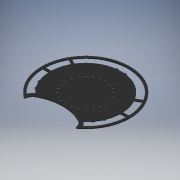
# Autodesk Inventor part: MotorPlate
Saved by Autodesk Inventor 2017 (Build 210142000, 142)
## iProperties
Created: 2019-01-31
Part Number: MotorPlate
Material: Generic
Document SubType Name: Modeling
Designer: cresswnd
Density: 1 g/cm^3
Appearance: Smooth - Black
Author: cresswnd
Autodesk Inventor part; units mm, degrees
ref_plane "YZ Plane" through (0, 0, 0) normal (1, 0, 0) x (0, 1, 0)
ref_plane "XZ Plane" through (0, 0, 0) normal (0, 1, 0) x (-1, 0, 0)
ref_plane "XY Plane" through (0, 0, 0) normal (0, 0, 1) x (1, 0, 0)
sketch "Sketch1" plane through (0, 0, 0) normal (0, 1, 0) x (-1, 0, 0)
  circle A0 centre (0, 0) radius 13.5 construction
  circle A1 centre (0, 0) radius 43
  line L0 (0, 0) -> (0, 137) construction
  line L1 (0, 43) -> (0, 47.5) construction
  circle A2 centre (0, 47.5) radius 2.5
  circle A3 centre (-6.2, 47.0936) radius 2.5
  circle A4 centre (-12.2939, 45.8815) radius 2.5
  circle A5 centre (-18.1775, 43.8843) radius 2.5
  circle A6 centre (-23.75, 41.1362) radius 2.5
  circle A7 centre (-28.9162, 37.6843) radius 2.5
  circle A8 centre (-33.5876, 33.5876) radius 2.5
  circle A9 centre (-37.6843, 28.9162) radius 2.5
  circle A10 centre (-41.1362, 23.75) radius 2.5
  circle A11 centre (-43.8843, 18.1775) radius 2.5
  circle A12 centre (-45.8815, 12.2939) radius 2.5
  circle A13 centre (-47.0936, 6.2) radius 2.5
  circle A14 centre (-47.5, 0) radius 2.5
  circle A15 centre (-47.0936, -6.2) radius 2.5
  circle A16 centre (-45.8815, -12.2939) radius 2.5
  circle A17 centre (-43.8843, -18.1775) radius 2.5
  circle A18 centre (-41.1362, -23.75) radius 2.5
  circle A19 centre (-37.6843, -28.9162) radius 2.5
  circle A20 centre (-33.5876, -33.5876) radius 2.5
  circle A21 centre (-28.9162, -37.6843) radius 2.5
  circle A22 centre (-23.75, -41.1362) radius 2.5
  circle A23 centre (-18.1775, -43.8843) radius 2.5
  circle A24 centre (-12.2939, -45.8815) radius 2.5
  circle A25 centre (-6.2, -47.0936) radius 2.5
  circle A26 centre (0, -47.5) radius 2.5
  circle A27 centre (6.2, -47.0936) radius 2.5
  circle A28 centre (12.2939, -45.8815) radius 2.5
  circle A29 centre (18.1775, -43.8843) radius 2.5
  circle A30 centre (23.75, -41.1362) radius 2.5
  circle A31 centre (28.9162, -37.6843) radius 2.5
  circle A32 centre (33.5876, -33.5876) radius 2.5
  circle A33 centre (37.6843, -28.9162) radius 2.5
  circle A34 centre (41.1362, -23.75) radius 2.5
  circle A35 centre (43.8843, -18.1775) radius 2.5
  circle A36 centre (45.8815, -12.2939) radius 2.5
  circle A37 centre (47.0936, -6.2) radius 2.5
  circle A38 centre (47.5, 0) radius 2.5
  circle A39 centre (47.0936, 6.2) radius 2.5
  circle A40 centre (45.8815, 12.2939) radius 2.5
  circle A41 centre (43.8843, 18.1775) radius 2.5
  circle A42 centre (41.1362, 23.75) radius 2.5
  circle A43 centre (37.6843, 28.9162) radius 2.5
  circle A44 centre (33.5876, 33.5876) radius 2.5
  circle A45 centre (28.9162, 37.6843) radius 2.5
  circle A46 centre (23.75, 41.1362) radius 2.5
  circle A47 centre (18.1775, 43.8843) radius 2.5
  circle A48 centre (12.2939, 45.8815) radius 2.5
  circle A49 centre (6.2, 47.0936) radius 2.5
  line L2 (0, 105) -> (0, 80) construction
  line L3 (0, 80) -> (-94, 80) construction
  line L4 (0, 80) -> (0, 55) construction
  line L5 (60, 80) -> (60, 65) construction
  line L6 (-60, 80) -> (-60, 65) construction
  line L7 (-60, 80) -> (-50, 80) construction
  line L8 (-50, 80) -> (-50, 65) construction
  line L9 (60, 80) -> (50, 80) construction
  line L10 (50, 80) -> (50, 65) construction
  arc A50 (-50, 67.6691) -> (50, 67.6691) centre (0, 160) ccw
  arc A51 (-60, 80) -> (-50, 67.6691) centre (-40.1315, 85.8924) ccw
  arc A52 (50, 67.6691) -> (60, 80) centre (40.1315, 85.8924) ccw
  circle A53 centre (-40.1315, 85.8924) radius 20.7239 construction
  circle A54 centre (40.1315, 85.8924) radius 20.7239 construction
  line L11 (0, 0) -> (0, -105) construction
  line L12 (0, 0) -> (105, 0) construction
  line L13 (0, 0) -> (105, 0) construction
  line L14 (0, 0) -> (-141, 0) construction
  line L15 (60, 0) -> (100, 0) construction
  line L16 (80, 0) -> (80, -2.5) construction
  line L17 (80, -2.5) -> (80, 2.5) construction
  line L18 (-60, 0) -> (-100, 0) construction
  line L19 (-80, 0) -> (-80, -2.5) construction
  line L20 (-80, -2.5) -> (-80, 2.5) construction
  line L21 (0, 0) -> (86.6025, 50) construction
  line L22 (0, 0) -> (100, 0) construction
  line L23 (0, 0) -> (-90.9327, 52.5) construction
  line L24 (0, 0) -> (105, 0) construction
  line L25 (-86.6025, 50) -> (-71.0141, 41) construction
  line L26 (-66.3266, 49.119) -> (-75.7016, 32.881) construction
  circle A55 centre (-66.3266, 49.119) radius 1.5 construction
  circle A56 centre (-66.3266, 49.119) radius 4 construction
  circle A57 centre (-75.7016, 32.881) radius 1.5 construction
  circle A58 centre (-75.7016, 32.881) radius 4 construction
  circle A59 centre (-75.7016, 32.881) radius 1.5
  circle A60 centre (-66.3266, 49.119) radius 1.5
  line L27 (71.0141, 41) -> (80.3891, 41) construction
  line L28 (66.3266, 49.119) -> (75.7016, 32.881) construction
  circle A61 centre (75.7016, 32.881) radius 1.5
  circle A62 centre (66.3266, 49.119) radius 1.5
  circle A63 centre (75.7016, 32.881) radius 4 construction
  circle A64 centre (66.3266, 49.119) radius 4 construction
  arc A65 (-73.8998, 29.3098) -> (-71.8618, 34.0019) centre (-75.7016, 32.881) ccw
  arc A66 (-76.0333, 36.8672) -> (-78.8412, 30.4025) centre (-75.7016, 32.881) ccw
  arc A67 (-65.75, 53.0772) -> (-69.9446, 47.4131) centre (-66.3266, 49.119) ccw
  arc A68 (-65.3774, 45.2332) -> (-62.3329, 49.3443) centre (-66.3266, 49.119) ccw
  arc A69 (62.3329, 49.3443) -> (65.3774, 45.2332) centre (66.3266, 49.119) ccw
  arc A70 (69.9446, 47.4131) -> (65.75, 53.0772) centre (66.3266, 49.119) ccw
  arc A71 (71.8618, 34.0019) -> (73.8998, 29.3098) centre (75.7016, 32.881) ccw
  arc A72 (78.8412, 30.4025) -> (76.0333, 36.8672) centre (75.7016, 32.881) ccw
  line L29 (9.375, -82) -> (-9.375, -82) construction
  circle A73 centre (-9.375, -82) radius 1.5
  circle A74 centre (9.375, -82) radius 1.5
  circle A75 centre (9.375, -82) radius 4 construction
  circle A76 centre (-9.375, -82) radius 4 construction
  arc A77 (6.0887, -84.2804) -> (13.0912, -83.4798) centre (9.375, -82) ccw
  arc A78 (11.5669, -78.654) -> (6.4844, -79.2351) centre (9.375, -82) ccw
  arc A79 (-13.0912, -83.4798) -> (-6.0887, -84.2804) centre (-9.375, -82) ccw
  arc A80 (-6.4844, -79.2351) -> (-11.5669, -78.654) centre (-9.375, -82) ccw
  line L30 (0, -60) -> (0, -100) construction
  line L31 (-2.5, -82) -> (2.5, -82) construction
  arc A81 (-47.8941, 66.5594) -> (47.8941, 66.5594) centre (0, 0) ccw construction
  arc A82 (60, 80) -> (60.8528, 85.5683) centre (40.1315, 85.8924) ccw
  arc A83 (-60.8528, 85.5683) -> (-60, 80) centre (-40.1315, 85.8924) ccw
  line L32 (0, 0) -> (90.9327, -52.5) construction
  line L33 (0, 0) -> (105, 0) construction
  line L34 (0, 0) -> (-90.9327, -52.5) construction
  line L35 (71.0141, -41) -> (69.7641, -43.1651) construction
  line L36 (71.0141, -41) -> (73.5141, -41) construction
  line L37 (69.7641, -43.1651) -> (72.2641, -38.8349) construction
  line L38 (72.2641, -38.8349) -> (97.3626, -38.8349) construction
  line L39 (-51.9615, 30) -> (-68.849, 39.75) construction
  line L40 (-60.4053, 34.875) -> (-61.6553, 32.7099) construction
  line L41 (-61.6553, 32.7099) -> (-59.1553, 37.0401) construction
  line L42 (-61.6553, 32.7099) -> (-50.6664, 26.3655) construction
  line L43 (-59.1553, 37.0401) -> (-46.9615, 30) construction
  line L44 (51.9615, 30) -> (68.849, 39.75) construction
  line L45 (60.4053, 34.875) -> (59.1553, 37.0401) construction
  line L46 (59.1553, 37.0401) -> (61.6553, 32.7099) construction
  line L47 (61.6553, 32.7099) -> (48.3013, 25) construction
  line L48 (59.1553, 37.0401) -> (44.9783, 28.855) construction
  arc A84 (59.4525, 64.4927) -> (29.303, 59.1718) centre (40.1315, 85.8924) ccw construction
  arc A85 (67.7078, 70.1562) -> (-67.7078, 70.1562) centre (0, 160) ccw construction
  arc A86 (30.4498, 51.6992) -> (51.925, 60.2) centre (0, 160) ccw
  arc A87 (56.5784, 62.7625) -> (59.4525, 64.4927) centre (0, 160) ccw
  arc A88 (-59.4525, 64.4927) -> (-56.5784, 62.7625) centre (0, 160) ccw
  arc A89 (-51.925, 60.2) -> (-30.4498, 51.6992) centre (0, 160) ccw
  arc A90 (-51.925, 60.2) -> (-62.3329, 49.3443) centre (0, 0) ccw
  arc A91 (-56.5784, 62.7625) -> (-65.75, 53.0772) centre (0, 0) ccw
  arc A92 (-65.3774, 45.2332) -> (-67.565, 41.8954) centre (0, 0) ccw
  line L49 (-50.6664, 32.139) -> (-67.565, 41.8954)
  line L50 (-53.1664, 27.8089) -> (-70.065, 37.5653)
  arc A93 (-70.065, 37.5653) -> (-71.8618, 34.0019) centre (0, 0) ccw
  arc A94 (-73.8998, 29.3098) -> (-79.4607, 2.5) centre (0, 0) ccw
  line L51 (-59.9479, -2.5) -> (-79.4607, -2.5)
  line L52 (-79.4607, 2.5) -> (-59.9479, 2.5)
  arc A95 (-79.4607, -2.5) -> (-70.065, -37.5653) centre (0, 0) ccw
  line L53 (-70.065, -37.5653) -> (-53.1664, -27.8089)
  line L54 (-67.565, -41.8954) -> (-50.6664, -32.139)
  arc A96 (-30.4498, 51.6992) -> (-50.6664, 32.139) centre (0, 0) ccw
  arc A97 (-53.1664, 27.8089) -> (-59.9479, 2.5) centre (0, 0) ccw
  arc A98 (65.75, 53.0772) -> (56.5784, 62.7625) centre (0, 0) ccw
  arc A99 (62.3329, 49.3443) -> (51.925, 60.2) centre (0, 0) ccw
  line L55 (50.6664, 32.139) -> (67.565, 41.8954)
  arc A100 (71.8971, 44.3966) -> (69.9446, 47.4131) centre (0, 0) ccw
  line L56 (53.1664, 27.8089) -> (70.065, 37.5653)
  arc A101 (67.565, 41.8954) -> (65.3774, 45.2332) centre (0, 0) ccw
  arc A102 (50.6664, 32.139) -> (30.4498, 51.6992) centre (0, 0) ccw
  arc A103 (76.0333, 36.8672) -> (74.3971, 40.0664) centre (0, 0) ccw
  arc A104 (71.8618, 34.0019) -> (70.065, 37.5653) centre (0, 0) ccw
  arc A105 (59.9479, 2.5) -> (53.1664, 27.8089) centre (0, 0) ccw
  arc A106 (84.463, 2.5) -> (78.8412, 30.4025) centre (0, 0) ccw
  arc A107 (79.4607, 2.5) -> (73.8998, 29.3098) centre (0, 0) ccw
  line L57 (79.4607, -2.5) -> (59.9479, -2.5)
  line L58 (59.9479, 2.5) -> (79.4607, 2.5)
  arc A108 (53.1664, -27.8089) -> (59.9479, -2.5) centre (0, 0) ccw
  arc A109 (70.065, -37.5653) -> (79.4607, -2.5) centre (0, 0) ccw
  line L59 (70.065, -37.5653) -> (53.1664, -27.8089)
  line L60 (72.2641, -38.8349) -> (72.2311, -38.8159)
  arc A110 (74.3971, -40.0664) -> (84.463, -2.5) centre (0, 0) ccw
  line L61 (69.7641, -43.1651) -> (69.7311, -43.146)
  line L62 (67.565, -41.8954) -> (50.6664, -32.139)
  arc A111 (2.5, -59.9479) -> (50.6664, -32.139) centre (0, 0) ccw
  line L63 (-2.5, -79.4607) -> (-2.5, -59.9479)
  line L64 (2.5, -79.4607) -> (2.5, -59.9479)
  arc A112 (2.5, -84.463) -> (6.0887, -84.2804) centre (0, 0) ccw
  arc A113 (13.0912, -83.4798) -> (71.8971, -44.3966) centre (0, 0) ccw
  arc A114 (2.5, -79.4607) -> (6.4844, -79.2351) centre (0, 0) ccw
  arc A115 (11.5669, -78.654) -> (67.565, -41.8954) centre (0, 0) ccw
  arc A116 (-71.8971, -44.3966) -> (-13.0912, -83.4798) centre (0, 0) ccw
  arc A117 (-6.0887, -84.2804) -> (-2.5, -84.463) centre (0, 0) ccw
  arc A118 (-67.565, -41.8954) -> (-11.5669, -78.654) centre (0, 0) ccw
  arc A119 (-6.4844, -79.2351) -> (-2.5, -79.4607) centre (0, 0) ccw
  arc A120 (-59.9479, -2.5) -> (-53.1664, -27.8089) centre (0, 0) ccw
  arc A121 (-50.6664, -32.139) -> (-2.5, -59.9479) centre (0, 0) ccw
  arc A122 (-60.8528, 85.5683) -> (60.8528, 85.5683) centre (0, 0) ccw
  arc A123 (74.3971, 40.0664) -> (71.8971, 44.3966) centre (0, 0) ccw
  arc A124 (-2.5, -84.463) -> (2.5, -84.463) centre (0, 0) ccw
  arc A125 (-78.8412, 30.4025) -> (-84.463, 2.5) centre (0, 0) ccw
  arc A126 (-84.463, -2.5) -> (-74.3971, -40.0664) centre (0, 0) ccw
  arc A127 (-59.4525, 64.4927) -> (-56.5784, 62.7625) centre (0, 160) ccw
  arc A128 (-69.9446, 47.4131) -> (-76.0333, 36.8672) centre (0, 0) ccw
  arc A129 (-29.303, 59.1718) -> (-47.4945, 58.017) centre (-40.1315, 85.8924) ccw construction
  arc A130 (59.4525, 64.4927) -> (66.6416, 74.5581) centre (40.1315, 85.8924) ccw
  arc A131 (-66.6416, 74.5581) -> (-59.4525, 64.4927) centre (-40.1315, 85.8924) ccw
  arc A132 (-66.6416, 74.5581) -> (66.6416, 74.5581) centre (0, 0) ccw
  arc A133 (-51.925, 60.2) -> (51.925, 60.2) centre (0, 160) ccw
  arc A134 (56.5784, 62.7625) -> (59.4525, 64.4927) centre (0, 160) ccw
  line L65 (71.8971, -44.3966) -> (85.3255, -52.1494)
  line L66 (71.8971, -44.3966) -> (87.4028, -44.3966) construction
  line L67 (74.3971, -40.0664) -> (87.8255, -47.8193)
  line L68 (74.3971, -40.0664) -> (89.9028, -40.0664) construction
  line L69 (84.463, -2.5) -> (99.9687, -2.5)
  line L70 (84.463, -2.5) -> (99.9687, -2.5) construction
  line L71 (84.463, 2.5) -> (99.9687, 2.5)
  line L72 (84.463, 2.5) -> (99.9687, 2.5) construction
  line L73 (-84.463, 2.5) -> (-99.9687, 2.5)
  line L74 (-84.463, 2.5) -> (-68.9573, 2.5) construction
  line L75 (-84.463, -2.5) -> (-99.9687, -2.5)
  line L76 (-84.463, -2.5) -> (-68.9573, -2.5) construction
  line L77 (-71.8971, -44.3966) -> (-85.3255, -52.1494)
  line L78 (-71.8971, -44.3966) -> (-56.3914, -44.3966) construction
  line L79 (-74.3971, -40.0664) -> (-87.8255, -47.8193)
  line L80 (-74.3971, -40.0664) -> (-58.8914, -40.0664) construction
  point P0 (-65.5107, 72.2122)
  dimension "d109" = 86
  dimension "d108" = 27
  dimension "d110" = 4.5
  dimension "d111" = 5
  dimension "d114" = 360
  dimension "d117" = 25
  dimension "d118" = 25
  dimension "d119" = 10
  dimension "d120" = 10
  dimension "d125" = 2.5
  dimension "d126" = 5
  dimension "d127" = 2.5
  dimension "d128" = 5
  dimension "d130" = 30
  dimension "d131" = 150
  dimension "d132" = 18
  dimension "d137" = 18.75
  dimension "d140" = 3
  dimension "d141" = 8
  dimension "d142" = 3
  dimension "d143" = 8
  dimension "d146" = 18.75
  dimension "d147" = 3
  dimension "d148" = 3
  dimension "d149" = 8
  dimension "d150" = 8
  dimension "d153" = 18.75
  dimension "d154" = 3
  dimension "d155" = 3
  dimension "d156" = 8
  dimension "d157" = 8
  dimension "d159" = 5
  dimension "d162" = 30
  dimension "d163" = 2.5
  dimension "d164" = 120
  dimension "d165" = 5
  dimension "d170" = 5
  dimension "d171" = 2.5
  dimension "d172" = 5
  dimension "d183" = 30
  dimension "d184" = 30
  dimension "d185" = 0
  dimension "d186" = 0
  dimension "d187" = 180
  dimension "d188" = 180
  dimension "d189" = 150
  dimension "d190" = 150
  constraints: 180 point on circle, 163 end point, 131 centre point, 31 point on line, 27 coincident, 18 horizontal, 12 equal length, 10 concentric, 6 vertical, 4 midpoint, 4 perpendicular, 3 tangent, 1 vertical alignment, 121 other
  measures "d108" diameter of A0
  measures "d110" distance of L1.start L1.end
  measures "d111" diameter of A2
  measures "d117" distance of L2.start L2.end
  measures "d118" distance of L2.end L4.end
  measures "d119" distance of L6.start L7.end
  measures "d120" distance of L5.start L9.end
  measures "d125" distance of L16.end L16.start
  measures "d126" distance of L16.end L17.end
  measures "d127" distance of L19.start L19.end
  measures "d128" distance of L20.end L19.end
  measures "d130" angle of L22 L21
  measures "d131" angle of L24 L23
  measures "d132" distance of L25.start L25.end
  measures "d137" distance of L26.start L26.end
  measures "d140" diameter of A55
  measures "d141" diameter of A56
  measures "d142" diameter of A57
  measures "d143" diameter of A58
  measures "d146" distance of L28.start L28.end
  measures "d147" diameter of A61
  measures "d148" diameter of A62
  measures "d149" diameter of A63
  measures "d150" diameter of A64
  measures "d153" distance of L29.start L29.end
  measures "d154" diameter of A73
  measures "d155" diameter of A74
  measures "d156" diameter of A75
  measures "d157" diameter of A76
  measures "d159" distance of L31.start L31.end
  measures "d162" angle of L32 L33
  measures "d163" distance of L35.start L35.end
  measures "d164" angle of L35 L36
  measures "d165" distance of L35.end L37.end
  measures "d170" distance of L40.end L41.end
  measures "d171" distance of L45.start L45.end
  measures "d172" distance of L45.end L46.end
  measures "d183" angle of L65 L66
  measures "d184" angle of L67 L68
  measures "d185" distance between parallel lines of L70 L69
  measures "d186" distance between parallel lines of L72 L71
  measures "d187" angle of L73 L74
  measures "d188" angle of L75 L76
  measures "d189" angle of L77 L78
  measures "d190" angle of L79 L80
extrude "Extrusion6" add sketch "Sketch1" along normal blind 2
fillet "Fillet7" radius 1 2 edges at (-60.8528, 1, 85.5683) (60.8528, 1, 85.5683)
sketch "Sketch4" plane through (0, 0, 0) normal (0, -1, 0) x (1, 0, 0)
  arc A0 (-79.4607, -2.5) -> (-70.065, -37.5653) centre (0, 0) ccw projected
  line L0 (-79.4607, -2.5) -> (-59.9479, -2.5) projected
  line L1 (-53.1664, -27.8089) -> (-70.065, -37.5653) projected
  arc A1 (-59.9479, -2.5) -> (-53.1664, -27.8089) centre (0, 0) ccw projected
  arc A2 (-73.8998, 29.3098) -> (-79.4607, 2.5) centre (0, 0) ccw projected
  arc A3 (-73.8998, 29.3098) -> (-71.8618, 34.0019) centre (-75.7016, 32.881) ccw projected
  arc A4 (-70.065, 37.5653) -> (-71.8618, 34.0019) centre (0, 0) ccw projected
  line L2 (-70.065, 37.5653) -> (-53.1664, 27.8089) projected
  arc A5 (-53.1664, 27.8089) -> (-59.9479, 2.5) centre (0, 0) ccw projected
  line L3 (-59.9479, 2.5) -> (-79.4607, 2.5) projected
  arc A6 (-65.3774, 45.2332) -> (-67.565, 41.8954) centre (0, 0) ccw projected
  line L4 (-50.6664, 32.139) -> (-67.565, 41.8954) projected
  arc A7 (-65.3774, 45.2332) -> (-62.3329, 49.3443) centre (-66.3266, 49.119) ccw projected
  arc A8 (-51.925, 60.2) -> (-62.3329, 49.3443) centre (0, 0) ccw projected
  arc A9 (-51.925, 60.2) -> (-30.4498, 51.6992) centre (0, 160) ccw projected
  arc A10 (-30.4498, 51.6992) -> (-50.6664, 32.139) centre (0, 0) ccw projected
  line L5 (59.9479, -2.5) -> (79.4607, -2.5) projected
  arc A11 (53.1664, -27.8089) -> (59.9479, -2.5) centre (0, 0) ccw projected
  line L6 (70.065, -37.5653) -> (53.1664, -27.8089) projected
  arc A12 (70.065, -37.5653) -> (79.4607, -2.5) centre (0, 0) ccw projected
  arc A13 (79.4607, 2.5) -> (73.8998, 29.3098) centre (0, 0) ccw projected
  line L7 (79.4607, 2.5) -> (59.9479, 2.5) projected
  arc A14 (59.9479, 2.5) -> (53.1664, 27.8089) centre (0, 0) ccw projected
  line L8 (53.1664, 27.8089) -> (70.065, 37.5653) projected
  arc A15 (71.8618, 34.0019) -> (70.065, 37.5653) centre (0, 0) ccw projected
  arc A16 (71.8618, 34.0019) -> (73.8998, 29.3098) centre (75.7016, 32.881) ccw projected
  arc A17 (67.565, 41.8954) -> (65.3774, 45.2332) centre (0, 0) ccw projected
  arc A18 (62.3329, 49.3443) -> (65.3774, 45.2332) centre (66.3266, 49.119) ccw projected
  arc A19 (62.3329, 49.3443) -> (51.925, 60.2) centre (0, 0) ccw projected
  arc A20 (30.4498, 51.6992) -> (51.925, 60.2) centre (0, 160) ccw projected
  arc A21 (50.6664, 32.139) -> (30.4498, 51.6992) centre (0, 0) ccw projected
  line L9 (67.565, 41.8954) -> (50.6664, 32.139) projected
extrude "Extrusion7" add sketch "Sketch4" against normal blind 2
fillet "Fillet8" radius 2 28 edges at (-85.3255, 1, -52.1494) (-67.565, 1, -41.8954) (-50.6664, 1, -32.139) (-2.5, 1, -59.9479) (-2.5, 1, -79.4607) (-71.8971, 1, -44.3966) (-84.463, 1, -2.5) (-66.6416, 1, 74.5581) (-99.9687, 1, -2.5) (-74.3971, 1, -40.0664) (-87.8255, 1, -47.8193) (85.3255, 1, -52.1494) (67.565, 1, -41.8954) (2.5, 1, -79.4607) (50.6664, 1, -32.139) (2.5, 1, -59.9479) (71.8971, 1, -44.3966) (87.8255, 1, -47.8193) (74.3971, 1, -40.0664) (99.9687, 1, -2.5) (84.463, 1, -2.5) (99.9687, 1, 2.5) (84.463, 1, 2.5) (56.5784, 1, 62.7625) (66.6416, 1, 74.5581) (-56.5784, 1, 62.7625) (-99.9687, 1, 2.5) (-84.463, 1, 2.5)
sketch "Sketch6" plane through (0, 2, 0) normal (0, 1, 0) x (1, 0, 0)
  arc A0 (84.2153, 53.9239) -> (-84.2153, 53.9239) centre (0, 0) ccw construction
  arc A1 (-88.8071, 45.9706) -> (-99.8945, 4.5918) centre (0, 0) ccw construction
  arc A2 (-84.2153, 53.9239) -> (-83.531, 51.1134) centre (-82.531, 52.8454) ccw construction
  line L0 (-88.8071, 45.9706) -> (-84.2153, 53.9239) construction
  line L1 (-86.5112, 49.9473) -> (-90.9327, 52.5) construction
  arc A3 (62.337, -84.4932) -> (-62.337, -84.4932) centre (0, 0) ccw construction
  line L2 (-86.5112, 49.9473) -> (-81.4057, 49.9473) construction
  line L3 (84.2153, 53.9239) -> (88.8071, 45.9706) construction
  line L4 (86.5112, 49.9473) -> (90.9327, 52.5) construction
  line L5 (86.5112, 49.9473) -> (91.6167, 49.9473) construction
  circle A4 centre (86.5112, 49.9473) radius 1.5
  circle A5 centre (-86.5112, 49.9473) radius 1.5
  dimension "d214" = 150
  dimension "d216" = 30
  dimension "d262" = 3
  dimension "d263" = 3
  constraints: 12 end point, 2 centre point, 2 coincident, 2 equal length, 2 horizontal, 2 midpoint, 2 point on circle
  measures "d214" angle of L2 L1
  measures "d216" angle of L5 L4
  measures "d262" diameter of A4
  measures "d263" diameter of A5
extrude "Extrusion9" cut sketch "Sketch6" against normal up to next
sketch "Sketch7" plane through (0, 2, 0) normal (0, 1, 0) x (1, 0, 0)
  circle A0 centre (6.2, -47.0936) radius 2.5 projected
  circle A1 centre (28.9162, -37.6843) radius 2.5 projected
  circle A2 centre (18.1775, -43.8843) radius 2.5 projected
  circle A3 centre (37.6843, -28.9162) radius 2.5 projected
  circle A4 centre (43.8843, -18.1775) radius 2.5 projected
  circle A5 centre (47.0936, -6.2) radius 2.5 projected
  circle A6 centre (47.0936, 6.2) radius 2.5 projected
  circle A7 centre (43.8843, 18.1775) radius 2.5 projected
  circle A8 centre (37.6843, 28.9162) radius 2.5 projected
  circle A9 centre (28.9162, 37.6843) radius 2.5 projected
  circle A10 centre (18.1775, 43.8843) radius 2.5 projected
  circle A11 centre (6.2, 47.0936) radius 2.5 projected
  circle A12 centre (-6.2, 47.0936) radius 2.5 projected
  circle A13 centre (-18.1775, 43.8843) radius 2.5 projected
  circle A14 centre (-28.9162, 37.6843) radius 2.5 projected
  circle A15 centre (-37.6843, 28.9162) radius 2.5 projected
  circle A16 centre (-43.8843, 18.1775) radius 2.5 projected
  circle A17 centre (-47.0936, 6.2) radius 2.5 projected
  circle A18 centre (-47.0936, -6.2) radius 2.5 projected
  circle A19 centre (-43.8843, -18.1775) radius 2.5 projected
  circle A20 centre (-37.6843, -28.9162) radius 2.5 projected
  circle A21 centre (-28.9162, -37.6843) radius 2.5 projected
  circle A22 centre (-18.1775, -43.8843) radius 2.5 projected
  circle A23 centre (-6.2, -47.0936) radius 2.5 projected
  circle A24 centre (6.2, -47.0936) radius 1.55
  circle A25 centre (18.1775, -43.8843) radius 1.55
  circle A26 centre (28.9162, -37.6843) radius 1.55
  circle A27 centre (37.6843, -28.9162) radius 1.55
  circle A28 centre (43.8843, -18.1775) radius 1.55
  circle A29 centre (47.0936, -6.2) radius 1.55
  circle A30 centre (47.0936, 6.2) radius 1.55
  circle A31 centre (43.8843, 18.1775) radius 1.55
  circle A32 centre (37.6843, 28.9162) radius 1.55
  circle A33 centre (28.9162, 37.6843) radius 1.55
  circle A34 centre (18.1775, 43.8843) radius 1.55
  circle A35 centre (6.2, 47.0936) radius 2.5 projected
  circle A36 centre (6.2, 47.0936) radius 1.55
  circle A37 centre (-6.2, 47.0936) radius 1.55
  circle A38 centre (-18.1775, 43.8843) radius 1.55
  circle A39 centre (-28.9162, 37.6843) radius 1.55
  circle A40 centre (-37.6843, 28.9162) radius 1.55
  circle A41 centre (-43.8843, 18.1775) radius 1.55
  circle A42 centre (-47.0936, 6.2) radius 1.55
  circle A43 centre (-47.0936, -6.2) radius 1.55
  circle A44 centre (-43.8843, -18.1775) radius 2.5 projected
  circle A45 centre (-43.8843, -18.1775) radius 1.55
  circle A46 centre (-37.6843, -28.9162) radius 1.55
  circle A47 centre (-28.9162, -37.6843) radius 1.55
  circle A48 centre (-18.1775, -43.8843) radius 1.55
  circle A49 centre (-6.2, -47.0936) radius 1.55
  point P0 (0, 0)
  dimension "d220" = 3.1
  dimension "d221" = 3.1
  dimension "d222" = 3.1
  dimension "d223" = 3.1
  dimension "d224" = 3.1
  dimension "d225" = 3.1
  dimension "d226" = 3.1
  dimension "d227" = 3.1
  dimension "d228" = 3.1
  dimension "d229" = 3.1
  dimension "d230" = 3.1
  dimension "d231" = 3.1
  dimension "d232" = 3.1
  dimension "d233" = 3.1
  dimension "d234" = 3.1
  dimension "d235" = 3.1
  dimension "d236" = 3.1
  dimension "d237" = 3.1
  dimension "d238" = 3.1
  dimension "d239" = 3.1
  dimension "d240" = 3.1
  dimension "d241" = 3.1
  dimension "d242" = 3.1
  dimension "d243" = 3.1
  constraints: 24 centre point, 24 coincident
  measures "d220" diameter of A24
  measures "d221" diameter of A25
  measures "d222" diameter of A26
  measures "d223" diameter of A27
  measures "d224" diameter of A28
  measures "d225" diameter of A29
  measures "d226" diameter of A30
  measures "d227" diameter of A31
  measures "d228" diameter of A32
  measures "d229" diameter of A33
  measures "d230" diameter of A34
  measures "d231" diameter of A36
  measures "d232" diameter of A37
  measures "d233" diameter of A38
  measures "d234" diameter of A39
  measures "d235" diameter of A40
  measures "d236" diameter of A41
  measures "d237" diameter of A42
  measures "d238" diameter of A43
  measures "d239" diameter of A45
  measures "d240" diameter of A46
  measures "d241" diameter of A47
  measures "d242" diameter of A48
  measures "d243" diameter of A49
extrude "Extrusion10" add sketch "Sketch7" against normal up to surface (2 mm away)
sketch "Sketch8" plane through (0, 0, 0) normal (0, -1, 0) x (1, 0, 0)
  circle A0 centre (0, 0) radius 43 projected
  circle A1 centre (-18.1775, 43.8843) radius 1.55 projected
  circle A2 centre (-6.2, 47.0936) radius 1.55 projected
  circle A3 centre (-28.9162, 37.6843) radius 1.55 projected
  circle A4 centre (-43.8843, 18.1775) radius 1.55 projected
  circle A5 centre (-47.0936, -6.2) radius 1.55 projected
  circle A6 centre (-37.6843, -28.9162) radius 1.55 projected
  circle A7 centre (-18.1775, -43.8843) radius 1.55 projected
  circle A8 centre (6.2, -47.0936) radius 1.55 projected
  circle A9 centre (28.9162, -37.6843) radius 1.55 projected
  circle A10 centre (43.8843, -18.1775) radius 1.55 projected
  circle A11 centre (47.0936, 6.2) radius 1.55 projected
  circle A12 centre (37.6843, 28.9162) radius 1.55 projected
  circle A13 centre (28.9162, 37.6843) radius 1.55 projected
  circle A14 centre (6.2, 47.0936) radius 1.55 projected
  circle A15 centre (18.1775, 43.8843) radius 1.55 projected
  circle A16 centre (43.8843, 18.1775) radius 1.55 projected
  circle A17 centre (47.0936, -6.2) radius 1.55 projected
  circle A18 centre (37.6843, -28.9162) radius 1.55 projected
  circle A19 centre (18.1775, -43.8843) radius 1.55 projected
  circle A20 centre (-6.2, -47.0936) radius 1.55 projected
  circle A21 centre (-28.9162, -37.6843) radius 1.55 projected
  circle A22 centre (-43.8843, -18.1775) radius 1.55 projected
  circle A23 centre (-47.0936, 6.2) radius 1.55 projected
  circle A24 centre (-37.6843, 28.9162) radius 1.55 projected
  circle A25 centre (0, 0) radius 43 projected
  line L0 (73.5598, -45.3565) -> (83.531, -51.1134) projected
  arc A26 (84.2153, -53.9239) -> (83.531, -51.1134) centre (82.531, -52.8454) ccw projected
  arc A27 (-84.2153, -53.9239) -> (84.2153, -53.9239) centre (0, 0) ccw projected
  arc A28 (-83.531, -51.1134) -> (-84.2153, -53.9239) centre (-82.531, -52.8454) ccw projected
  line L1 (-83.531, -51.1134) -> (-73.5598, -45.3565) projected
  arc A29 (-70.8821, -45.9998) -> (-73.5598, -45.3565) centre (-72.5598, -47.0885) ccw projected
  arc A30 (-70.8821, -45.9998) -> (-13.0912, -83.4798) centre (0, 0) ccw projected
  arc A31 (-13.0912, -83.4798) -> (-6.0887, -84.2804) centre (-9.375, -82) ccw projected
  arc A32 (-6.0887, -84.2804) -> (6.0887, -84.2804) centre (0, 0) ccw projected
  arc A33 (6.0887, -84.2804) -> (13.0912, -83.4798) centre (9.375, -82) ccw projected
  arc A34 (13.0912, -83.4798) -> (70.8821, -45.9998) centre (0, 0) ccw projected
  arc A35 (73.5598, -45.3565) -> (70.8821, -45.9998) centre (72.5598, -47.0885) ccw projected
  arc A36 (11.5669, -78.654) -> (66.4248, -43.6806) centre (0, 0) ccw projected
  arc A37 (11.5669, -78.654) -> (6.4844, -79.2351) centre (9.375, -82) ccw projected
  arc A38 (4.6161, -79.3659) -> (6.4844, -79.2351) centre (0, 0) ccw projected
  arc A39 (2.5, -77.3692) -> (4.6161, -79.3659) centre (4.5, -77.3692) ccw projected
  line L2 (2.5, -77.3692) -> (2.5, -61.8365) projected
  arc A40 (4.3548, -59.8418) -> (2.5, -61.8365) centre (4.5, -61.8365) ccw projected
  arc A41 (4.3548, -59.8418) -> (49.6471, -33.6923) centre (0, 0) ccw projected
  arc A42 (52.302, -33.0833) -> (49.6471, -33.6923) centre (51.302, -34.8154) ccw projected
  line L3 (52.302, -33.0833) -> (65.7537, -40.8497) projected
  arc A43 (66.4248, -43.6806) -> (65.7537, -40.8497) centre (64.7537, -42.5817) ccw projected
  arc A44 (-6.4844, -79.2351) -> (-4.6161, -79.3659) centre (0, 0) ccw projected
  arc A45 (-6.4844, -79.2351) -> (-11.5669, -78.654) centre (-9.375, -82) ccw projected
  arc A46 (-66.4248, -43.6806) -> (-11.5669, -78.654) centre (0, 0) ccw projected
  arc A47 (-65.7537, -40.8497) -> (-66.4248, -43.6806) centre (-64.7537, -42.5817) ccw projected
  line L4 (-65.7537, -40.8497) -> (-52.302, -33.0833) projected
  arc A48 (-49.6471, -33.6923) -> (-52.302, -33.0833) centre (-51.302, -34.8154) ccw projected
  arc A49 (-49.6471, -33.6923) -> (-4.3548, -59.8418) centre (0, 0) ccw projected
  arc A50 (-2.5, -61.8365) -> (-4.3548, -59.8418) centre (-4.5, -61.8365) ccw projected
  line L5 (-2.5, -61.8365) -> (-2.5, -77.3692) projected
  arc A51 (-4.6161, -79.3659) -> (-2.5, -77.3692) centre (-4.5, -77.3692) ccw projected
  arc A52 (78.8412, 30.4025) -> (76.0333, 36.8672) centre (75.7016, 32.881) ccw projected
  arc A53 (76.0333, 36.8672) -> (69.9446, 47.4131) centre (0, 0) ccw projected
  arc A54 (69.9446, 47.4131) -> (65.75, 53.0772) centre (66.3266, 49.119) ccw projected
  arc A55 (65.75, 53.0772) -> (58.5062, 60.9694) centre (0, 0) ccw projected
  arc A56 (58.8449, 64.1171) -> (58.5062, 60.9694) centre (59.891, 62.4125) ccw projected
  arc A57 (58.8449, 64.1171) -> (59.4525, 64.4927) centre (0, 160) ccw projected
  arc A58 (59.4525, 64.4927) -> (65.511, 72.2128) centre (40.1315, 85.8924) ccw projected
  arc A59 (68.6444, 72.7182) -> (65.511, 72.2128) centre (67.2715, 71.2639) ccw projected
  arc A60 (99.8945, 4.5918) -> (68.6444, 72.7182) centre (0, 0) ccw projected
  arc A61 (97.8966, 2.5) -> (99.8945, 4.5918) centre (97.8966, 4.5) ccw projected
  line L6 (97.8966, 2.5) -> (86.3829, 2.5) projected
  arc A62 (84.3856, 4.396) -> (86.3829, 2.5) centre (86.3829, 4.5) ccw projected
  arc A63 (84.3856, 4.396) -> (78.8412, 30.4025) centre (0, 0) ccw projected
  line L7 (-86.3829, 2.5) -> (-97.8966, 2.5) projected
  arc A64 (-99.8945, 4.5918) -> (-97.8966, 2.5) centre (-97.8966, 4.5) ccw projected
  arc A65 (-68.6444, 72.7182) -> (-99.8945, 4.5918) centre (0, 0) ccw projected
  arc A66 (-65.511, 72.2128) -> (-68.6444, 72.7182) centre (-67.2715, 71.2639) ccw projected
  arc A67 (-65.511, 72.2128) -> (-59.4525, 64.4927) centre (-40.1315, 85.8924) ccw projected
  arc A68 (-59.4525, 64.4927) -> (-58.8449, 64.1171) centre (0, 160) ccw projected
  arc A69 (-58.5062, 60.9694) -> (-58.8449, 64.1171) centre (-59.891, 62.4125) ccw projected
  arc A70 (-58.5062, 60.9694) -> (-65.75, 53.0772) centre (0, 0) ccw projected
  arc A71 (-65.75, 53.0772) -> (-69.9446, 47.4131) centre (-66.3266, 49.119) ccw projected
  arc A72 (-69.9446, 47.4131) -> (-76.0333, 36.8672) centre (0, 0) ccw projected
  arc A73 (-76.0333, 36.8672) -> (-78.8412, 30.4025) centre (-75.7016, 32.881) ccw projected
  arc A74 (-78.8412, 30.4025) -> (-84.3856, 4.396) centre (0, 0) ccw projected
  arc A75 (-86.3829, 2.5) -> (-84.3856, 4.396) centre (-86.3829, 4.5) ccw projected
  line L8 (86.3829, -2.5) -> (97.8966, -2.5) projected
  arc A76 (99.8945, -4.5918) -> (97.8966, -2.5) centre (97.8966, -4.5) ccw projected
  arc A77 (88.8071, -45.9706) -> (99.8945, -4.5918) centre (0, 0) ccw projected
  arc A78 (86.031, -46.7833) -> (88.8071, -45.9706) centre (87.031, -45.0512) ccw projected
  line L9 (86.031, -46.7833) -> (76.0598, -41.0264) projected
  arc A79 (75.278, -38.3858) -> (76.0598, -41.0264) centre (77.0598, -39.2943) ccw projected
  arc A80 (75.278, -38.3858) -> (84.3856, -4.396) centre (0, 0) ccw projected
  arc A81 (86.3829, -2.5) -> (84.3856, -4.396) centre (86.3829, -4.5) ccw projected
  line L10 (-76.0598, -41.0264) -> (-86.031, -46.7833) projected
  arc A82 (-88.8071, -45.9706) -> (-86.031, -46.7833) centre (-87.031, -45.0512) ccw projected
  arc A83 (-99.8945, -4.5918) -> (-88.8071, -45.9706) centre (0, 0) ccw projected
  arc A84 (-97.8966, -2.5) -> (-99.8945, -4.5918) centre (-97.8966, -4.5) ccw projected
  line L11 (-97.8966, -2.5) -> (-86.3829, -2.5) projected
  arc A85 (-84.3856, -4.396) -> (-86.3829, -2.5) centre (-86.3829, -4.5) ccw projected
  arc A86 (-84.3856, -4.396) -> (-75.278, -38.3858) centre (0, 0) ccw projected
  arc A87 (-76.0598, -41.0264) -> (-75.278, -38.3858) centre (-77.0598, -39.2943) ccw projected
  circle A88 centre (-12.2939, 45.8815) radius 2.5 projected
  circle A89 centre (-23.75, 41.1362) radius 2.5 projected
  circle A90 centre (-33.5876, 33.5876) radius 2.5 projected
  circle A91 centre (-41.1362, 23.75) radius 2.5 projected
  circle A92 centre (-45.8815, 12.2939) radius 2.5 projected
  circle A93 centre (-47.5, 0) radius 2.5 projected
  circle A94 centre (-45.8815, -12.2939) radius 2.5 projected
  circle A95 centre (-41.1362, -23.75) radius 2.5 projected
  circle A96 centre (-33.5876, -33.5876) radius 2.5 projected
  circle A97 centre (-23.75, -41.1362) radius 2.5 projected
  circle A98 centre (-12.2939, -45.8815) radius 2.5 projected
  circle A99 centre (0, -47.5) radius 2.5 projected
  circle A100 centre (12.2939, -45.8815) radius 2.5 projected
  circle A101 centre (23.75, -41.1362) radius 2.5 projected
  circle A102 centre (33.5876, -33.5876) radius 2.5 projected
  circle A103 centre (41.1362, -23.75) radius 2.5 projected
  circle A104 centre (45.8815, -12.2939) radius 2.5 projected
  circle A105 centre (47.5, 0) radius 2.5 projected
  circle A106 centre (45.8815, 12.2939) radius 2.5 projected
  circle A107 centre (41.1362, 23.75) radius 2.5 projected
  circle A108 centre (33.5876, 33.5876) radius 2.5 projected
  circle A109 centre (23.75, 41.1362) radius 2.5 projected
  circle A110 centre (12.2939, 45.8815) radius 2.5 projected
  circle A111 centre (0, 47.5) radius 2.5 projected
  circle A112 centre (-9.375, -82) radius 1.5 projected
  circle A113 centre (9.375, -82) radius 1.5 projected
  circle A114 centre (-66.3266, 49.119) radius 1.5 projected
  circle A115 centre (-75.7016, 32.881) radius 1.5 projected
  circle A116 centre (66.3266, 49.119) radius 1.5 projected
  circle A117 centre (75.7016, 32.881) radius 1.5 projected
  arc A118 (62.337, 84.4932) -> (60.7484, 83.79) centre (61.7433, 83.6885) ccw projected
  arc A119 (50, 67.6691) -> (60.7484, 83.79) centre (40.1315, 85.8924) ccw projected
  arc A120 (-50, 67.6691) -> (50, 67.6691) centre (0, 160) ccw projected
  arc A121 (-60.7484, 83.79) -> (-50, 67.6691) centre (-40.1315, 85.8924) ccw projected
  arc A122 (-60.7484, 83.79) -> (-62.337, 84.4932) centre (-61.7433, 83.6885) ccw projected
  arc A123 (-62.337, 84.4932) -> (62.337, 84.4932) centre (0, 0) ccw projected
extrude "Extrusion11" add sketch "Sketch8" against normal blind 2 contours A0 | A37 A38 A39 L2 A40 A41 A42 L3 A43 A36 | A45 A46 A47 L4 A48 A49 A50 L5 A51 A44
sketch "Sketch10" plane through (0, 2, 0) normal (0, 1, 0) x (1, 0, 0)
  circle A0 centre (-18.1775, 43.8843) radius 1.55 projected
  circle A1 centre (18.1775, 43.8843) radius 1.55 projected
  line L0 (-18.1775, 43.8843) -> (-18.1775, 35.3843) construction
  circle A2 centre (-18.1775, 35.3843) radius 1.5
  line L1 (18.1775, 43.8843) -> (18.1775, 35.3843) construction
  circle A3 centre (18.1775, 35.3843) radius 1.5
  point P0 (0, 0)
  point P1 (47.5, 0)
  point P2 (-47.5, 0)
  dimension "d252" = 8.5
  dimension "d253" = 3
  dimension "d254" = 8.5
  dimension "d255" = 3
  constraints: 4 end point, 2 centre point, 2 coincident, 2 vertical
  measures "d252" distance of L0.start L0.end
  measures "d253" diameter of A2
  measures "d254" distance of L1.start L1.end
  measures "d255" diameter of A3
extrude "Extrusion14" cut sketch "Sketch10" against normal up to next
body "Solid6"
